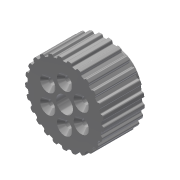
# Autodesk Inventor part: Synchronous Pulley1
Saved by Autodesk Inventor 2018 (Build 220112000, 112)
## iProperties
CustomPartVersion: 1
Created: 2020-03-19
Part Number: Synchronous Pulley1
Material: Steel
Document SubType Name: Modeling
Designer: Bunny320
Density: 1 g/cm^3
Appearance: Steel
Author: Bunny320
## iProperties of the stored document Synchronous Pulley1_3DPrint.ipt
Created: 2020-05-08
Part Number: Synchronous Pulley1_3DPrint
Material: Generic
Document SubType Name: Modeling
Designer: Bunny320
Density: 1 g/cm^3
Appearance: Default
Author: Bunny320
Autodesk Inventor part; units mm, degrees
ref_plane "YZ Plane" through (0, 0, 0) normal (1, 0, 0) x (0, 1, 0)
ref_plane "XZ Plane" through (0, 0, 0) normal (0, 1, 0) x (-1, 0, 0)
ref_plane "XY Plane" through (0, 0, 0) normal (0, 0, 1) x (1, 0, 0)
sketch "Pulley Sketch" plane through (0, 0, 0) normal (0, 0, 1) x (1, 0, 0)
  circle A0 centre (0, 0) radius 19.8944 construction
  circle A1 centre (0, 0) radius 19.3944
  circle A2 centre (0, 0) radius 18.1444
  line L0 (-1.4573, 19.3395) -> (-0.9, 18.1444)
  line L1 (-0.9, 18.1444) -> (0.9, 18.1444)
  line L2 (0.9, 18.1444) -> (1.4573, 19.3395)
  line L3 (0, 0) -> (0, 19.3944) construction
  point P0 (0, 18.1444)
  dimension "d0" = 39.7887
  dimension "d1" = 0.5
  dimension "d2" = 1.25
  dimension "d3" = 50
  dimension "d4" = 1.8
  constraints: 8 end point, 3 coincident, 3 point on circle, 2 centre point, 1 horizontal, 1 midpoint, 1 point on line, 1 vertical, 1 vertical alignment, 3 other
  measures "d0" diameter of A0
  measures "d1" radial gap between concentric circles of A0 A1
  measures "d3" angle of L2 L0
  measures "d4" distance of L0.end L1.end
extrude "Base Body" add sketch "Pulley Sketch" along normal mid plane 20 contours A2 | A1 L0 L1 L2 | L2 L1 L0 A1
extrude "Tooth" cut sketch "Pulley Sketch" along normal through all both and the other way through all contours L2 L1 L0 A1 picked at (0, 18.9737)
fillet "Tooth Fillet" radius 0.4 2 edges at (0.9, 18.1444, 0) (-0.9, 18.1444, 0)
fillet "Tooth Fillet" radius 0.6 4 edges at (-1.4573, 19.3395, 5) (-1.4573, 19.3395, -5) (1.4573, 19.3395, 5) (1.4573, 19.3395, -5)
sketch "Sketch3" plane through (0, 0, 10) normal (0, 0, 1) x (1, 0, 0)
  circle A0 centre (0, 0) radius 16
  dimension "d20" = 32
  constraints: 1 centre point, 1 coincident
  measures "d20" diameter of A0
sketch "Sketch4" plane through (0, 0, 6) normal (0, 0, 1) x (1, 0, 0)
  circle A0 centre (0, 0) radius 15.5
  dimension "d23" = 31
  constraints: 1 centre point, 1 coincident
  measures "d23" diameter of A0
pattern_circular "Teeth" count 25 over 360 about axis through (0, 0, -10) along (0, 0, 1) of "Tooth", "Tooth Fillet"
feature "Left flange" [suppressed]
feature "Right flange" [suppressed]
sketch "Sketch2" plane through (0, 0, 0) normal (0, 0, 1) x (1, 0, 0)
  circle A0 centre (0, 0) radius 12.7
  dimension "d17" = 25.4
  constraints: 1 centre point, 1 coincident
  measures "d17" diameter of A0
extrude "Extrusion3" add sketch "Sketch2" against normal blind 15
sketch "Sketch5" plane through (0, 0, -15) normal (0, 0, -1) x (-1, 0, 0)
  circle A0 centre (0, 0) radius 4.15
  line L0 (-1.5, 3.1) -> (1.5, 3.1)
  line L1 (1.5, 3.1) -> (1.5, 5.2)
  line L2 (1.5, 5.2) -> (-1.5, 5.2)
  line L3 (-1.5, 5.2) -> (-1.5, 3.1)
  line L4 (-1.5, 3.1) -> (1.5, 5.2) construction
  line L5 (1.5, 3.1) -> (-1.5, 5.2) construction
  point P0 (0, 4.15)
  point P1 (0, 4.15)
  dimension "d26" = 8.3
  dimension "d27" = 3
  dimension "d28" = 5.2
  constraints: 12 end point, 3 midpoint, 2 parallel, 2 vertical alignment, 1 coincident, 1 horizontal, 1 perpendicular, 2 other
  measures "d27" distance of L1.end L2.end
  measures "d28" distance from line of point (0, 0) L2
extrude "Extrusion6" cut sketch "Sketch5" against normal through all contours A0 L3 L0 L1 | L1 L0 L3 A0
sketch "Sketch6" plane through (0, 0, 10) normal (0, 0, 1) x (1, 0, 0)
  point P0 (0, 0)
  point P1 (0, 9.525)
  dimension "d31" = 9.525
  constraints: 1 vertical alignment
  measures "d31" distance of point (0, 0) point (0, 9.525)
hole "Hole1" at (0, 9.525, 10) direction (0, 0, -1) diameter 3.4 end through all countersink diameter 7.5 countersink angle 90 clearance for "Countersunk Flat Head Hex Socket Screw DIN EN ISO 10642" size "M3" standard "DIN"
pattern_circular "Circular Pattern2" count 6 over 360 about axis through (0, 0, -10) along (0, 0, 1) of "Hole1"
chamfer "Chamfer1" distance 1 angle 45 1 edges at (4.15, 0, -15)
equation "\"d1\" = da_a"
equation "\"d2\" = da_hg"
equation "\"d3\" = 2 * da_fi"
equation "\"d4\" = da_bw"
equation "\"d5\" = da_bf"
equation "\"d7\" = da_bf"
equation "\"d9\" = da_rb"
equation "\"d10\" = da_rt"
equation "\"da_pb\" = 5"
equation "\"da_fi\" = 25deg"
equation "\"da_hg\" = 1.25"
equation "\"da_bw\" = 1.8"
equation "\"da_rb\" = 0.4"
equation "\"da_rt\" = 0.6"
equation "\"da_a\" = 0.5"
equation "\"da_bf\" = 20"
equation "\"da_wf\" = 1"
equation "\"da_hf\" = 1.2"
body "Solid1"
